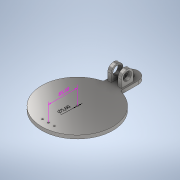
# Autodesk Inventor part: Base do telescópio
Saved by Autodesk Inventor 2021 (Build 250183000, 183)
## iProperties
Created: 2021-08-10
Part Number: Base do telescópio
Material: Steel, Carbon
Document SubType Name: Modeling
Designer: guilh
Density: 7.85 g/cm^3
Appearance: Semi-Polished
Author: guilh
Autodesk Inventor part; units mm, degrees
ref_plane "YZ Plane" through (0, 0, 0) normal (1, 0, 0) x (0, 1, 0)
ref_plane "XZ Plane" through (0, 0, 0) normal (0, 1, 0) x (-1, 0, 0)
ref_plane "XY Plane" through (0, 0, 0) normal (0, 0, 1) x (1, 0, 0)
sketch "Sketch1" plane through (0, 0, 0) normal (0, 1, 0) x (-1, 0, 0)
  circle A0 centre (0, 0) radius 105
  dimension "d0" = 210
  constraints: 1 centre point, 1 coincident
  measures "d0" diameter of A0
extrude "Extrusion1" add sketch "Sketch1" along normal blind 10
sketch "Sketch2" plane through (0, 10, 0) normal (0, 1, 0) x (1, 0, 0)
  line L0 (-79.8594, -68.6516) -> (79.5179, -68.6516)
  line L1 (0, 0) -> (0, -80)
  line L2 (0, -80) -> (0, -60)
  line L3 (0, -60) -> (17.5, -60)
  line L4 (0, -60) -> (-17.5, -60)
  circle A0 centre (-17.5, -60) radius 2.5
  circle A1 centre (0, -60) radius 2.5
  circle A2 centre (17.5, -60) radius 2.5
  dimension "d4" = 80
  dimension "d5" = 20
  dimension "d6" = 17.5
  dimension "d7" = 17.5
  dimension "d8" = 5
  dimension "d9" = 5
  dimension "d10" = 5
  constraints: 10 end point, 3 centre point, 3 coincident, 2 horizontal, 1 perpendicular, 1 point on line, 1 vertical
  measures "d4" distance of L1.start L1.end
  measures "d5" distance of L1.end L2.end
  measures "d6" distance of L2.end L3.end
  measures "d7" distance of L2.end L4.end
  measures "d8" diameter of A0
  measures "d9" diameter of A1
  measures "d10" diameter of A2
extrude "Extrusion2" cut sketch "Sketch2" against normal blind 10
sketch "Sketch3" plane through (0, 10, 0) normal (0, 1, 0) x (1, 0, 0)
  circle A0 centre (0, 0) radius 2.5
  dimension "d13" = 5
  constraints: 1 centre point, 1 coincident
  measures "d13" diameter of A0
extrude "Extrusion3" cut sketch "Sketch3" against normal blind 10
sketch "Sketch4" plane through (0, 10, 0) normal (0, 1, 0) x (1, 0, 0)
  circle A0 centre (0, 0) radius 2.5 projected
  line L0 (0, 0) -> (0, 80)
  line L1 (-15, 80) -> (-15, 65)
  line L2 (-15, 65) -> (15, 65)
  line L3 (15, 65) -> (15, 95)
  line L4 (15, 95) -> (-15, 95)
  line L5 (-15, 95) -> (-15, 80)
  line L6 (0, 80) -> (-7.5, 80)
  line L7 (-7.5, 80) -> (7.5, 80)
  line L8 (7.5, 80) -> (7.5, 95)
  line L9 (7.5, 80) -> (7.5, 65)
  line L10 (-7.5, 80) -> (-7.5, 95)
  line L11 (-7.5, 80) -> (-7.5, 65)
  dimension "d20" = 15
  dimension "d21" = 15
  dimension "d22" = 30
  dimension "d23" = 30
  dimension "d24" = 7.5
  dimension "d25" = 15
  constraints: 24 end point, 8 point on line, 5 perpendicular, 1 horizontal, 1 vertical
  measures "d20" distance of L0.end L1.start
  measures "d21" distance of L1.start L1.end
  measures "d22" distance of L1.end L2.end
  measures "d23" distance of L2.end L3.end
  measures "d24" distance of L0.end L6.end
  measures "d25" distance of L6.end L7.end
extrude "Extrusion4" add sketch "Sketch4" along normal blind 30 contours L2 L11 L6 L0 | L0 L7 L9 L2 | L6 L10 L4 L8 L7
sketch "Sketch5" plane through (7.5, 10, -65) normal (1, 0, 0) x (0, 0, -1)
  line L0 (40, 0) -> (-170, 0) projected
  line L1 (40, 0) -> (15, 0)
  line L2 (15, 0) -> (15, 15)
  circle A0 centre (15, 15) radius 7.5
  line L3 (30, 0) -> (30, 30) projected
  arc A1 (30, 15) -> (0, 15) centre (15, 15) ccw
  line L4 (15, 15) -> (0, 15) construction
  line L5 (15, 15) -> (30, 15) construction
  line L6 (0, 0) -> (0, 30) projected
  line L7 (0, 15) -> (0, 30)
  line L8 (0, 30) -> (30, 30) projected
  line L9 (0, 30) -> (30, 30)
  line L10 (30, 30) -> (30, 15)
  point P0 (-65, -10)
  point P1 (15, 30)
  dimension "d28" = 25
  dimension "d29" = 15
  dimension "d30" = 15
  dimension "d31" = 180
  constraints: 14 end point, 2 centre point, 2 coincident, 2 perpendicular, 2 point on circle, 1 collinear, 1 midpoint, 1 point on line
  measures "d28" distance of L0.start L1.end
  measures "d29" distance of L1.end L2.end
  measures "d30" diameter of A0
  measures "d31" angle of L4 L5
extrude "Extrusion5" cut sketch "Sketch5" against normal blind 30 contours A1 L8 L3 | A1 L6 L8 | A0
sketch "Sketch6" plane through (7.5, 10, -65) normal (1, 0, 0) x (0, 0, -1)
  circle A0 centre (15, 15) radius 7.5 projected
  circle A1 centre (15, 15) radius 5
  circle A2 centre (15, 15) radius 7.5
  point P0 (-65, -10)
  dimension "d34" = 10
  constraints: 2 centre point, 2 coincident
  measures "d34" diameter of A1
extrude "Extrusion6" add sketch "Sketch6" against normal blind 15
sketch "Sketch7" plane through (7.5, 10, -65) normal (1, 0, 0) x (0, 0, -1)
  line L0 (0, 0) -> (30, 0) projected
  line L1 (0, 0) -> (30, 0)
  line L2 (30, 0) -> (30, 34.6991)
  line L3 (30, 34.6991) -> (0, 34.6991)
  line L4 (0, 34.6991) -> (0, 0)
  point P0 (-65, -10)
  constraints: 8 end point, 3 perpendicular, 1 collinear
extrude "Extrusion7" cut sketch "Sketch7" against normal blind 15
sketch "Sketch8" plane through (0, 10, 0) normal (0, 1, 0) x (1, 0, 0)
  circle A0 centre (0, 0) radius 2.5 projected
  line L0 (0, 0) -> (0, 100)
  line L1 (0, 100) -> (-10, 100)
  line L2 (-10, 100) -> (-20, 100)
  line L3 (-20, 100) -> (-20, 65)
  line L4 (-20, 65) -> (-10, 65)
  line L5 (-10, 65) -> (-10, 100)
  line L6 (0, 100) -> (10, 100)
  line L7 (10, 100) -> (20, 100)
  line L8 (20, 100) -> (20, 65)
  line L9 (20, 65) -> (10, 65)
  line L10 (10, 65) -> (10, 100)
  dimension "d42" = 100
  dimension "d43" = 10
  dimension "d44" = 10
  dimension "d45" = 35
  dimension "d46" = 10
  dimension "d47" = 10
  dimension "d48" = 35
  constraints: 22 end point, 5 perpendicular, 5 point on line, 1 vertical
  measures "d42" distance of L0.start L0.end
  measures "d43" distance of L0.end L1.end
  measures "d44" distance of L1.end L2.end
  measures "d45" distance of L2.end L3.end
  measures "d46" distance of L0.end L6.end
  measures "d47" distance of L6.end L7.end
  measures "d48" distance of L7.end L8.end
extrude "Extrusion8" add sketch "Sketch8" along normal blind 35 contours L5 L4 L3 L2 | L7 L8 L9 L10
thicken "Thicken1" operation add thickness 5 both sides no extend neighbours yes toward (0, 1, 0) faces at (13.3333, 45, -88.3333)
thicken "Thicken2" operation add thickness 5 both sides no extend neighbours yes toward (0, 1, 0) faces at (-16.6667, 45, -88.3333)
sketch "Sketch10" plane through (20, 10, -65) normal (1, 0, 0) x (0, 0, -1)
  line L0 (0, 0) -> (35, 0) projected
  line L1 (0, 0) -> (17.5, 0)
  line L2 (17.5, 0) -> (17.5, 22.5)
  circle A0 centre (17.5, 22.5) radius 12.5
  circle A1 centre (17.5, 22.5) radius 17.5
  line L3 (35, 0) -> (35, 40) projected
  line L4 (0, 0) -> (0, 40) projected
  line L5 (0, 22.5) -> (0, 40)
  line L6 (35, 40) -> (0, 40) projected
  line L7 (0, 40) -> (35, 40)
  line L8 (35, 40) -> (35, 22.5)
  point P0 (-65, -10)
  point P1 (17.5, 40)
  dimension "d60" = 22.5
  dimension "d61" = 25
  constraints: 10 end point, 2 centre point, 2 coincident, 2 perpendicular, 2 point on circle, 2 point on line, 2 tangent, 1 collinear, 1 midpoint
  measures "d60" distance of L1.end L2.end
  measures "d61" diameter of A0
extrude "Extrusion9" cut sketch "Sketch10" against normal blind 40 contours L4 L6 A1 | L6 L3 A1 | A0
sketch "Sketch11" plane through (20, 10, -65) normal (1, 0, 0) x (0, 0, -1)
  line L0 (40, 0) -> (-170, 0) projected
  line L1 (35.2175, 0) -> (0.2175, 0)
  line L2 (0.2175, 0) -> (-34.7825, 0)
  line L3 (0.2175, 0) -> (40.2175, 0)
  circle A0 centre (40.2175, 17.5) radius 12.5
  circle A1 centre (40.2175, 17.5) radius 17.5
  line L4 (-34.7825, 0) -> (32.4725, 33.1928)
  point P0 (-65, -10)
  dimension "d73" = 35
  dimension "d74" = 35
  dimension "d75" = 40
  dimension "d78" = 35
  constraints: 8 end point, 3 point on line, 1 centre point, 1 coincident, 4 other
  measures "d73" distance of L1.start L1.end
  measures "d74" distance of L1.end L2.end
  measures "d75" distance of L3.start L3.end
  measures "d78" distance of L3.start L4.start
sketch "Sketch12" plane through (-20, 10, -100) normal (-1, 0, 0) x (0, 0, 1)
  line L0 (205, 0) -> (-5, 0) projected
  line L1 (37.401, 0) -> (37.401, 45.2729)
  line L2 (37.401, 45.2729) -> (-3.1543, 48.8051)
  line L3 (-3.1543, 48.8051) -> (-3.1543, 0)
  line L4 (37.401, 0) -> (-3.1543, 0)
  point P0 (100, -10)
  constraints: 8 end point, 2 point on line, 1 parallel, 1 perpendicular, 1 vertical
extrude "Extrusion10" cut sketch "Sketch12" against normal blind 40
extrude "Extrusion11" add sketch "Sketch11" against normal blind 40
sketch "Sketch13" plane through (0, 0, 0) normal (0, 0, 1) x (1, 0, 0)
  line L0 (105, 10) -> (-105, 10) projected
  line L1 (0, 10) -> (10, 10)
  line L2 (10, 10) -> (10, 48.8421)
  line L3 (20, 43.1928) -> (-20, 43.1928) projected
  line L4 (10, 48.8421) -> (-10, 48.8421)
  line L5 (-10, 48.8421) -> (-10, 10)
  line L6 (-10, 10) -> (10, 10)
  point P0 (0, 0)
  point P1 (-20, 10)
  point P2 (20, 10)
  dimension "d83" = 10
  dimension "d84" = 20
  constraints: 10 end point, 4 perpendicular, 2 point on line, 1 midpoint
  measures "d83" distance of L1.start L1.end
  measures "d84" distance of L2.end L4.end
extrude "Extrusion12" cut sketch "Sketch13" against normal blind 150
sketch "Sketch14" plane through (20, 10, -65) normal (1, 0, 0) x (0, 0, -1)
  line L0 (38.0776, 0) -> (-34.7825, 0) projected
  line L1 (-34.7825, 0) -> (42.8397, 49.7383)
  line L2 (42.8397, 49.7383) -> (77.8644, 0)
  line L3 (77.8644, 0) -> (-34.7825, 0)
  point P0 (-65, -10)
  constraints: 6 end point, 1 collinear
extrude "Extrusion13" cut sketch "Sketch14" against normal blind 150
sketch "Sketch15" plane through (0, 10, 0) normal (0, 1, 0) x (1, 0, 0)
  circle A0 centre (0, 0) radius 2.5 projected
  line L0 (0, 0) -> (0, 100)
  line L1 (0, 100) -> (-20, 100)
  line L2 (-20, 100) -> (-20, 65)
  line L3 (-20, 65) -> (-10, 65)
  line L4 (-10, 65) -> (-10, 100)
  line L5 (-10, 65) -> (10, 65)
  line L6 (10, 65) -> (20, 65)
  line L7 (20, 65) -> (20, 100)
  line L8 (20, 100) -> (10, 100)
  line L9 (10, 100) -> (10, 65)
  dimension "d89" = 100
  dimension "d90" = 20
  dimension "d91" = 35
  dimension "d92" = 10
  dimension "d93" = 20
  dimension "d94" = 10
  dimension "d95" = 35
  dimension "d96" = 10
  constraints: 20 end point, 4 point on line, 3 perpendicular, 1 midpoint, 1 vertical
  measures "d89" distance of L0.start L0.end
  measures "d90" distance of L0.end L1.end
  measures "d91" distance of L1.end L2.end
  measures "d92" distance of L2.end L3.end
  measures "d93" distance of L3.end L5.end
  measures "d94" distance of L5.end L6.end
  measures "d95" distance of L6.end L7.end
  measures "d96" distance of L7.end L8.end
extrude "Extrusion14" add sketch "Sketch15" along normal blind 40 contours L3 L2 L1 L4 | L9 L8 L7 L6
sketch "Sketch16" plane through (20, 10, -65) normal (1, 0, 0) x (0, 0, -1)
  line L0 (0, 40) -> (35, 40) projected
  line L1 (17.5, 40) -> (17.5, 22.5)
  circle A0 centre (17.5, 22.5) radius 12.5
  circle A1 centre (17.5, 22.5) radius 17.5
  line L2 (35, 0) -> (35, 40) projected
  line L3 (0, 0) -> (0, 40) projected
  line L4 (0, 22.5) -> (0, 40)
  line L5 (0, 40) -> (35, 40)
  line L6 (35, 40) -> (35, 22.5)
  point P0 (-65, -10)
  dimension "d99" = 17.5
  dimension "d100" = 25
  constraints: 8 end point, 2 centre point, 2 coincident, 2 point on circle, 2 point on line, 2 tangent, 1 collinear, 1 midpoint, 1 perpendicular, 1 vertical
  measures "d99" distance of L1.start L1.end
  measures "d100" diameter of A0
extrude "Extrusion15" cut sketch "Sketch16" against normal blind 40 contours L0 A1 L3 | L0 L2 A1 | A0
sketch "Sketch17" plane through (0, 10, 0) normal (0, 1, 0) x (1, 0, 0)
  line L0 (10, 100) -> (20, 100) projected
  line L1 (20, 100) -> (20, 150)
  line L2 (20, 150) -> (-20, 150)
  line L3 (-20, 65) -> (-20, 100) projected
  line L4 (-20, 150) -> (-20, 100)
  line L5 (-20, 100) -> (20, 100)
  point P0 (0, 0)
  dimension "d115" = 50
  dimension "d116" = 40
  constraints: 8 end point, 1 perpendicular, 1 vertical
  measures "d115" distance of L0.end L1.end
  measures "d116" distance of L1.end L2.end
extrude "Extrusion16" add sketch "Sketch17" against normal blind 10
sketch "Sketch18" plane through (0, 10, 0) normal (0, 1, 0) x (1, 0, 0)
  arc A0 (20, 130) -> (-20, 130) centre (0, 130) ccw projected
  circle A1 centre (0, 130) radius 10
  point P0 (0, 0)
  dimension "d120" = 20
  constraints: 1 centre point, 1 coincident
  measures "d120" diameter of A1
sketch "Sketch19" plane through (0, 10, 0) normal (0, 1, 0) x (1, 0, 0)
  arc A0 (-20, 103.0776) -> (20, 103.0776) centre (0, 0) ccw projected
  line L0 (0, -105) -> (0, -85)
  line L1 (24.5635, -53.4105) -> (22.0201, -67.8674)
  line L2 (22.0201, -67.8674) -> (-35.0046, -64.6548)
  line L3 (-35.0046, -64.6548) -> (-32.0998, -48.1432)
  line L4 (-32.0998, -48.1432) -> (24.5635, -53.4105)
  circle A1 centre (0, -85) radius 2.5
  circle A2 centre (17.5, -85) radius 2.5
  circle A3 centre (-17.5, -85) radius 2.5
  point P0 (-33.6, 99.4788)
  point P1 (33.6, 99.4788)
  dimension "d121" = 20
  dimension "d122" = 5
  dimension "d123" = 5
  dimension "d124" = 5
  constraints: 10 end point, 3 centre point, 1 coincident, 1 parallel, 1 point on circle, 1 vertical
  measures "d121" distance of L0.start L0.end
  measures "d122" diameter of A1
  measures "d123" diameter of A2
  measures "d124" diameter of A3
extrude "Extrusion17" cut sketch "Sketch19" against normal blind 10 contours A1 | A2 | A3
sketch "Sketch20" plane through (0, 10, 0) normal (0, 1, 0) x (1, 0, 0)
  line L0 (26.8391, -52.4734) -> (21.3508, -72.5526)
  line L1 (21.3508, -72.5526) -> (-28.5793, -65.8595)
  line L2 (-28.5793, -65.8595) -> (-28.5793, -48.1154)
  line L3 (-28.5793, -48.1154) -> (26.8391, -52.4734)
  point P0 (0, 0)
  constraints: 8 end point, 1 vertical
extrude "Extrusion18" add sketch "Sketch20" against normal blind 10
extrude "Extrusion19" cut sketch "Sketch18" against normal blind 10
sketch "Sketch22" plane through (0, 10, 0) normal (0, 1, 0) x (1, 0, 0)
  arc A0 (-33.6, 99.4788) -> (-20, 118.4272) centre (-40, 118.4272) ccw projected
  line L0 (0, 120.0651) -> (-25, 120.0651)
  line L1 (-25, 120.0651) -> (-25, 95.0651)
  line L2 (-25, 95.0651) -> (25, 95.0651)
  line L3 (25, 95.0651) -> (25, 120.0651)
  circle A1 centre (0, 130) radius 10 projected
  line L4 (0, 130) -> (0, 145)
  line L5 (0, 145) -> (0, 175)
  line L6 (0, 175) -> (-25, 175)
  line L7 (-25, 175) -> (-25, 120.0651)
  line L8 (0, 175) -> (25, 175)
  line L9 (25, 175) -> (25, 120.0651)
  line L10 (0, 145) -> (0, 155)
  circle A2 centre (0, 155) radius 10
  circle A3 centre (0, 155) radius 25
  point P0 (0, 0)
  point P1 (25, 155)
  point P2 (-25, 155)
  dimension "d137" = 25
  dimension "d138" = 25
  dimension "d139" = 50
  dimension "d140" = 25
  dimension "d141" = 15
  dimension "d142" = 30
  dimension "d143" = 25
  dimension "d144" = 10
  constraints: 22 end point, 3 perpendicular, 3 point on line, 2 coincident, 2 collinear, 2 vertical, 1 centre point, 1 horizontal, 1 tangent, 1 vertical alignment, 2 other
  measures "d137" distance of L0.start L0.end
  measures "d138" distance of L0.end L1.end
  measures "d139" distance of L1.end L2.end
  measures "d140" distance of L2.end L3.end
  measures "d141" distance of L4.start L4.end
  measures "d142" distance of L4.end L5.end
  measures "d143" distance of L5.end L6.end
  measures "d144" distance of L4.end L10.end
extrude "Extrusion20" add sketch "Sketch22" against normal blind 10 contours A1 A3 L9 L3 L2 L1 L0 | L0 L7 A3 A1 | A1 A3 | A3 L6 L5 A2 L4 A1 | A1 L4 A3 | L4 A2 L5 L8 A3 A1 | A1 A3 L4 | A3 L8 L6
fillet "Fillet2" radius 5 2 edges at (25, 5, -101.9804) (-25, 5, -101.9804)
sketch "Sketch23" plane through (0, 10, 0) normal (0, 1, 0) x (1, 0, 0)
  arc A0 (8.6603, 150) -> (-8.6603, 150) centre (0, 155) ccw projected
  circle A1 centre (0, 155) radius 10
  point P0 (0, 0)
  point P1 (-8.6603, 150)
  point P2 (8.6603, 150)
  constraints: 1 centre point, 1 coincident
extrude "Extrusion21" cut sketch "Sketch23" against normal blind 10
sketch "Sketch24" plane through (0, 10, 0) normal (0, 1, 0) x (1, 0, 0)
  line L0 (4.3067, 53.4932) -> (-39.3643, 61.3509)
  line L1 (-39.3643, 61.3509) -> (-15.7911, 128.1418)
  line L2 (-15.7911, 128.1418) -> (38.1554, 86.5864)
  line L3 (38.1554, 86.5864) -> (25.311, 39.7421)
  line L4 (25.311, 39.7421) -> (4.3067, 53.4932)
  point P0 (0, 0)
  constraints: 10 end point
extrude "Extrusion22" cut sketch "Sketch24" along normal blind 40
sketch "Sketch25" plane through (0, 10, 0) normal (0, 1, 0) x (1, 0, 0)
  circle A0 centre (0, 155) radius 10 projected
  line L0 (-10, 145) -> (-20, 145)
  line L1 (-20, 145) -> (-20, 110)
  line L2 (-20, 110) -> (-10, 110)
  line L3 (-10, 110) -> (-10, 145)
  line L4 (10, 145) -> (20, 145)
  line L5 (20, 145) -> (20, 110)
  line L6 (20, 110) -> (10, 110)
  line L7 (10, 110) -> (10, 145)
  point P0 (0, 0)
  dimension "d153" = 10
  dimension "d154" = 35
  dimension "d155" = 10
  dimension "d157" = 10
  constraints: 16 end point, 4 perpendicular, 3 point on line
  measures "d153" distance of L0.start L0.end
  measures "d154" distance of L0.end L1.end
  measures "d155" distance of L1.end L2.end
  measures "d157" distance of L4.start L4.end
extrude "Extrusion23" add sketch "Sketch25" along normal blind 40 contours L3 L2 L1 L0 | L4 L5 L6 L7
fillet "Fillet3" radius 17.5 4 edges at (15, 50, -110) (-15, 50, -110) (-15, 50, -145) (15, 50, -145)
sketch "Sketch26" plane through (20, 10, -110) normal (1, 0, 0) x (0, 0, -1)
  arc A0 (35, 22.5) -> (0, 22.5) centre (17.5, 22.5) ccw projected
  circle A1 centre (17.5, 22.5) radius 12.5
  point P0 (-110, -10)
  dimension "d161" = 25
  constraints: 1 centre point, 1 coincident
  measures "d161" diameter of A1
extrude "Extrusion24" cut sketch "Sketch26" against normal blind 40
body "Solid1"
